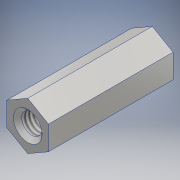
# Autodesk Inventor part: 18mm Standoff
Saved by Autodesk Inventor 2016 (Build 200138000, 138)
## iProperties
Created: 2016-05-23
Part Number: 18mm Standoff
Material: Aluminum 6061
Document SubType Name: Modeling
Designer: kromm.je.s
Density: 2.7 g/cm^3
Appearance: Aluminum - Flat
Author: kromm.je.s
Autodesk Inventor part; units mm, degrees
ref_plane "YZ Plane" through (0, 0, 0) normal (1, 0, 0) x (0, 1, 0)
ref_plane "XZ Plane" through (0, 0, 0) normal (0, 1, 0) x (-1, 0, 0)
ref_plane "XY Plane" through (0, 0, 0) normal (0, 0, 1) x (1, 0, 0)
sketch "Sketch1" plane through (0, 0, 0) normal (0, 1, 0) x (-1, 0, 0)
  line L0 (0, 0) -> (2.5, 0)
  line L1 (2.5, -1.4434) -> (0, -2.8868)
  line L2 (0, -2.8868) -> (-2.5, -1.4434)
  line L3 (-2.5, -1.4434) -> (-2.5, 1.4434)
  line L4 (-2.5, 1.4434) -> (0, 2.8868)
  line L5 (0, 2.8868) -> (2.5, 1.4434)
  line L6 (2.5, 1.4434) -> (2.5, -1.4434)
  dimension "d0" = 2.5
  constraints: 14 end point, 1 coincident, 1 horizontal, 1 midpoint, 13 other
  measures "d0" distance of L0.start L0.end
extrude "Extrusion1" add sketch "Sketch1" along normal blind 15
sketch "Sketch2" plane through (0, 15, 0) normal (0, 1, 0) x (1, 0, 0)
  point P0 (0, 0)
hole "Hole1" at (0, 15, 0) direction (0, -1, 0) diameter 2.459 end through all thread size "M3x0.5" class "6H" standard "ANSI Metric M Profile"
chamfer "Chamfer1" distance 0.5 angle 45 2 edges at (0, 15, -1.2295) (0, 0, -1.2295)
body "Solid1"
